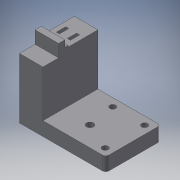
# Autodesk Inventor part: FixedFiber
Saved by Autodesk Inventor 2019 (Build 230136000, 136)
## iProperties
Created: 2019-06-10
Part Number: FixedFiber
Material: Generic
Document SubType Name: Modeling
Designer: aorfi
Density: 1 g/cm^3
Appearance: Default
Author: aorfi
Autodesk Inventor part; units mm, degrees
ref_plane "YZ Plane" through (0, 0, 0) normal (1, 0, 0) x (0, 1, 0)
ref_plane "XZ Plane" through (0, 0, 0) normal (0, 1, 0) x (-1, 0, 0)
ref_plane "XY Plane" through (0, 0, 0) normal (0, 0, 1) x (1, 0, 0)
sketch "Sketch1" plane through (0, 0, 0) normal (0, 1, 0) x (-1, 0, 0)
  line L0 (-27.5, 17.5) -> (27.5, 17.5)
  line L1 (27.5, 17.5) -> (27.5, -17.5)
  line L2 (27.5, -17.5) -> (-27.5, -17.5)
  line L3 (-27.5, -17.5) -> (-27.5, 17.5)
  line L4 (-27.5, 17.5) -> (27.5, -17.5) construction
  line L5 (27.5, 17.5) -> (-27.5, -17.5) construction
  point P0 (0, 0)
  dimension "d0" = 35
  dimension "d1" = 55
  constraints: 12 end point, 2 midpoint, 2 parallel, 1 horizontal, 1 perpendicular
  measures "d0" distance of L0.end L1.end
  measures "d1" distance of L1.end L2.end
extrude "Extrusion1" add sketch "Sketch1" along normal mid plane 8.763
sketch "Sketch2" plane through (0, 4.3815, 0) normal (0, 1, 0) x (1, 0, 0)
  line L0 (-27.5, -17.5) -> (27.5, -17.5) projected
  line L1 (27.5, -17.5) -> (27.5, 17.5) projected
  point P0 (4.8, -4.8)
  dimension "d11" = 12.7
  dimension "d12" = 22.7
  measures "d11" distance from line of L0 point (4.8, -4.8)
  measures "d12" distance from line of L1 point (4.8, -4.8)
hole "Hole1" at (4.8, 4.3815, 4.8) direction (0, -1, 0) diameter 4.496 end through all clearance for "Flat Head Machine Screw (82)" size "#8" standard "Ansi Unified Screw Threads"
sketch "Sketch3" plane through (0, 4.3815, 0) normal (0, 1, 0) x (1, 0, 0)
  line L0 (27.5, 17.5) -> (-27.5, 17.5) projected
  line L1 (-27.5, 17.5) -> (-12.5, 17.5)
  line L2 (-12.5, 17.5) -> (-12.5, -17.5)
  line L3 (-12.5, -17.5) -> (-27.5, -17.5)
  line L4 (-27.5, -17.5) -> (-27.5, 17.5)
  line L5 (-27.5, -17.5) -> (27.5, -17.5) projected
  point P0 (0, 0)
  dimension "d13" = 15
  constraints: 8 end point, 2 parallel, 1 collinear, 1 horizontal, 1 perpendicular
  measures "d13" distance of L2.end L3.end
extrude "Extrusion2" add sketch "Sketch3" along normal blind 32.66
sketch "Sketch4" plane through (0, 37.0415, 0) normal (0, 1, 0) x (1, 0, 0)
  line L0 (-12.5, -17.5) -> (-12.5, 17.5) projected
  line L1 (-27.5, -3.5) -> (-12.5, -3.5)
  line L2 (-12.5, -3.5) -> (-12.5, -7.5)
  line L3 (-12.5, -7.5) -> (-27.5, -7.5)
  line L4 (-27.5, -7.5) -> (-27.5, -3.5)
  line L5 (-27.5, 17.5) -> (-27.5, -17.5) projected
  line L6 (-27.5, -3.5) -> (-12.5, -3.5) construction
  line L7 (-12.5, -3.5) -> (-12.5, 3.5) construction
  line L8 (-12.5, 3.5) -> (-27.5, 3.5) construction
  line L9 (-27.5, 3.5) -> (-27.5, -3.5) construction
  line L10 (-27.5, -17.5) -> (-27.5, 17.5) construction
  line L11 (-27.5, 0) -> (-12.5, 0) construction
  line L12 (-27.5, -17.5) -> (-12.5, -17.5) projected
  point P0 (0, 0)
  dimension "d16" = 4
  dimension "d32" = 10
  constraints: 18 end point, 4 parallel, 4 point on line, 3 horizontal, 2 collinear, 2 midpoint, 2 perpendicular
  measures "d16" distance between parallel lines of L3 L1
  measures "d32" distance between parallel lines of L12 L3
extrude "Extrusion3" add sketch "Sketch4" along normal blind 5 contours L3 L4 L1 L0
sketch "Sketch5" plane through (0, 37.0415, 0) normal (0, 1, 0) x (1, 0, 0)
  line L0 (-24.5, 9) -> (-22.5, 9)
  line L1 (-22.5, 9) -> (-22.5, 3)
  line L2 (-22.5, 3) -> (-24.5, 3)
  line L3 (-24.5, 3) -> (-24.5, 9)
  line L4 (-15.5, 9) -> (-17.5, 9)
  line L5 (-17.5, 9) -> (-17.5, 3)
  line L6 (-17.5, 3) -> (-15.5, 3)
  line L7 (-15.5, 3) -> (-15.5, 9)
  line L8 (-23.5, 6) -> (-16.5, 6) construction
  line L9 (-12.5, -3.5) -> (-27.5, -3.5) construction
  line L10 (-7.5, 11.5) -> (-7.5, 1.5) construction
  line L11 (-7.5, 1.5) -> (-22.5, 1.5) construction
  line L12 (-27.5, 17.5) -> (-27.5, -3.5) construction
  line L13 (-27.5, -17.5) -> (-27.5, 17.5) construction
  point P0 (0, 0)
  point P1 (-20, -3.5)
  point P2 (-20, 6)
  point P3 (-16.5, 9)
  point P4 (-23.5, 9)
  point P5 (-22.5, 6)
  dimension "d20" = 6
  dimension "d21" = 2
  dimension "d22" = 5
  dimension "d26" = 1.5
  dimension "d31" = 7
  constraints: 22 end point, 5 midpoint, 4 parallel, 3 horizontal, 3 point on line, 3 vertical alignment, 2 perpendicular, 1 collinear
  measures "d20" distance of L2.end L0.start
  measures "d21" distance of L0.start L0.end
  measures "d22" distance between parallel lines of L9 L11
  measures "d26" distance between parallel lines of L2 L11
  measures "d31" distance of L8.start L8.end
extrude "Extrusion4" cut sketch "Sketch5" against normal blind 3
sketch "Sketch7" plane through (-27.5, -4.3815, -17.5) normal (-1, 0, 0) x (0, 0, 1)
  line L0 (35, 41.423) -> (25, 41.423)
  line L1 (25, 41.423) -> (25, 38.423)
  line L2 (25, 38.423) -> (35, 38.423)
  line L3 (35, 38.423) -> (35, 41.423)
  line L4 (25, 41.423) -> (25, 46.423) projected
  point P0 (17.5, 4.3815)
  dimension "d33" = 3
  constraints: 8 end point, 2 parallel, 1 collinear, 1 horizontal, 1 perpendicular
  measures "d33" distance between parallel lines of L2 L0
extrude "Extrusion6" cut sketch "Sketch7" against normal through all
sketch "Sketch8" plane through (0, 37.0415, 0) normal (0, 1, 0) x (1, 0, 0)
  line L0 (-27.5, -3.5) -> (-27, -3.5)
  line L1 (-27, -3.5) -> (-27, -1.5)
  line L2 (-27, -1.5) -> (-27.5, -1.5)
  line L3 (-27.5, -1.5) -> (-27.5, -3.5)
  line L4 (-12.5, -3.5) -> (-27.5, -3.5) projected
  line L5 (-27.5, 17.5) -> (-27.5, -3.5) projected
  point P0 (0, 0)
  dimension "d55" = 0.5
  dimension "d56" = 2
  constraints: 8 end point, 2 collinear, 2 parallel, 1 horizontal, 1 perpendicular
  measures "d55" distance of L2.end L1.end
  measures "d56" distance of L0.end L1.end
extrude "Extrusion7" add sketch "Sketch8" along normal blind 1
sketch "Sketch9" plane through (0, -4.3815, 0) normal (0, -1, 0) x (1, 0, 0)
  circle A0 centre (4.8, 4.8) radius 2.248 projected
  circle A1 centre (4.8, 4.8) radius 4
  point P0 (0, 0)
  dimension "d40" = 8
  constraints: 1 centre point, 1 coincident
  measures "d40" diameter of A1
extrude "Extrusion8" cut sketch "Sketch9" against normal blind 4.318
sketch "Sketch10" plane through (0, -4.3815, 0) normal (0, -1, 0) x (1, 0, 0)
  line L0 (27.5, -17.5) -> (27.5, 17.5) projected
  line L1 (-27.5, -17.5) -> (27.5, -17.5) projected
  point P0 (0, 0)
  point P1 (22.42, -12.42)
  point P2 (22.42, 12.726)
  point P3 (2.1, -12.42)
  dimension "d43" = 5.08
  dimension "d44" = 5.08
  dimension "d45" = 20.32
  dimension "d46" = 25.146
  constraints: 1 horizontal alignment, 1 vertical alignment
  measures "d43" distance from line of L0 point (22.42, -12.42)
  measures "d44" distance from line of L1 point (22.42, -12.42)
  measures "d45" distance of point (2.1, -12.42) point (22.42, -12.42)
  measures "d46" distance of point (22.42, -12.42) point (22.42, 12.726)
hole "Hole2" at (22.42, -4.3815, -12.42) at (22.42, -4.3815, 12.726) at (2.1, -4.3815, -12.42) direction (0, 1, 0) diameter 3.797 end through all clearance for "Flat Head Machine Screw (82)" size "#6" standard "Ansi Unified Screw Threads"
fillet "Fillet1" radius 2 2 edges at (27.5, 0, 17.5) (27.5, 0, -17.5)
equation "\"d44\" = d43"
body "Solid1"
